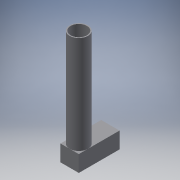
# Autodesk Inventor part: Part102
Saved by Autodesk Inventor 2016 (Build 200138000, 138)
## iProperties
Created: 2016-09-06
Part Number: Part102
Material: ABS Plastic
Document SubType Name: Modeling
Designer: gus
Density: 1.06 g/cm^3
Appearance: Smooth - White
Author: gus
Autodesk Inventor part; units mm, degrees
ref_plane "YZ Plane" through (0, 0, 0) normal (1, 0, 0) x (0, 1, 0)
ref_plane "XZ Plane" through (0, 0, 0) normal (0, 1, 0) x (-1, 0, 0)
ref_plane "XY Plane" through (0, 0, 0) normal (0, 0, 1) x (1, 0, 0)
sketch "Sketch1" plane through (0, 0, 0) normal (0, 1, 0) x (-1, 0, 0)
  circle A0 centre (0, 0) radius 28.575
  circle A1 centre (0, 0) radius 25.4
  dimension "d0" = 50.8
  dimension "d1" = 3.175
  constraints: 2 centre point, 2 coincident
  measures "d0" diameter of A1
  measures "d1" radial gap between concentric circles of A1 A0
extrude "Extrusion1" add sketch "Sketch1" along normal blind 304.8
sketch "Sketch2" plane through (0, 0, 0) normal (0, 1, 0) x (-1, 0, 0)
  line L0 (-28.575, 28.575) -> (28.575, 28.575)
  line L1 (28.575, 28.575) -> (28.575, -98.425)
  line L2 (28.575, -98.425) -> (-28.575, -98.425)
  line L3 (-28.575, -98.425) -> (-28.575, 28.575)
  circle A0 centre (0, 0) radius 28.575 projected
  dimension "d4" = 127
  constraints: 8 end point, 3 tangent, 2 parallel, 1 horizontal, 1 perpendicular
  measures "d4" distance between parallel lines of L2 L0
extrude "Extrusion2" add sketch "Sketch2" against normal blind 50.8
chamfer "Chamfer1" distance 68.2625 angle 4 1 edges at (0, 0, -98.425) measured on face at (0, 0, -97.925)
fillet "Fillet1" radius 19.05 10 edges at (28.575, -50.8, -34.925) (28.575, -27.7867, -98.425) (0, -4.7734, -98.425) (-28.575, -27.7867, -98.425) (0, -50.8, -98.425) (28.575, -25.4, 28.575) (0, -50.8, 28.575) (-28.575, -25.4, 28.575) (14.2875, 0, 28.575) (-14.2875, 0, 28.575)
sketch "Sketch3" plane through (-28.575, 0, -30.1625) normal (0, 0.9975641, -0.0697565) x (1, 0, 0)
  line L0 (0, 0) -> (57.15, 0) projected
  line L1 (38.1, 0) -> (22.225, 0)
  line L2 (22.225, 0) -> (22.225, 25.4)
  line L3 (22.225, 25.4) -> (38.1, 25.4)
  line L4 (38.1, 25.4) -> (38.1, 0)
  line L5 (38.1, 12.7) -> (22.225, 12.7)
  point P0 (28.575, -30.089)
  dimension "d11" = 15.875
  dimension "d12" = 25.4
  dimension "d13" = 9.525
  constraints: 10 end point, 2 midpoint, 2 parallel, 1 horizontal, 1 perpendicular, 1 point on line
  measures "d11" distance of L2.end L3.end
  measures "d12" distance of L1.end L2.end
  measures "d13" distance from line of point (28.575, -30.089) L4
revolve "Revolution1" add sketch "Sketch3" angle 100 about axis through (-28.575, 0, -30.1625) along (1, 0, 0) contours L2 L3 L4 L5
body "Solid1"
